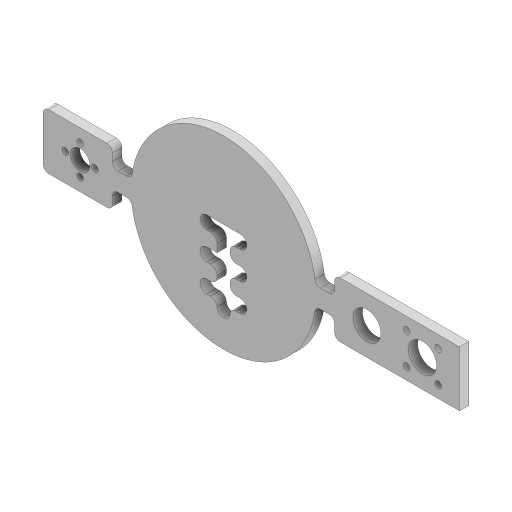
# Autodesk Inventor part: NUEVA TAPA PARA CORTE
Saved by Autodesk Inventor 2024 (Build 280153000, 153)
## iProperties
Created: 2024-05-26
Part Number: NUEVA TAPA PARA CORTE
Material: Generic
Document SubType Name: Modeling
Designer: Jhuliams
Density: 1 g/cm^3
Appearance: Default
Author: Jhuliams
Autodesk Inventor part; units mm, degrees
ref_plane "YZ Plane" through (0, 0, 0) normal (1, 0, 0) x (0, 1, 0)
ref_plane "XZ Plane" through (0, 0, 0) normal (0, 1, 0) x (-1, 0, 0)
ref_plane "XY Plane" through (0, 0, 0) normal (0, 0, 1) x (1, 0, 0)
sketch "Sketch1" plane through (0, 0, 0) normal (0, 0, 1) x (1, 0, 0)
  circle A0 centre (0, 0) radius 50
  line L0 (0, 0) -> (0, 20) construction
  line L1 (2.5, 15) -> (97.5, 15)
  line L2 (97.5, 15) -> (97.5, -15)
  line L3 (97.5, -15) -> (2.5, -15)
  line L4 (2.5, -15) -> (2.5, 15)
  line L5 (2.5, 15) -> (97.5, -15) construction
  line L6 (97.5, 15) -> (2.5, -15) construction
  line L7 (40, 5) -> (60, 5)
  line L8 (60, 5) -> (60, -5)
  line L9 (60, -5) -> (40, -5)
  line L10 (40, -5) -> (40, 5)
  line L11 (40, 5) -> (60, -5) construction
  line L12 (60, 5) -> (40, -5) construction
  line L13 (60, 5) -> (60, 15)
  line L14 (60, -5) -> (60, -15)
  line L15 (-2.5, 15) -> (-97.5, 15)
  line L16 (-97.5, 15) -> (-97.5, -15)
  line L17 (-97.5, -15) -> (-2.5, -15)
  line L18 (-2.5, -15) -> (-2.5, 15)
  line L19 (-2.5, 15) -> (-97.5, -15) construction
  line L20 (-97.5, 15) -> (-2.5, -15) construction
  line L21 (-40, 5) -> (-60, 5)
  line L22 (-60, 5) -> (-60, -5)
  line L23 (-60, -5) -> (-40, -5)
  line L24 (-40, -5) -> (-40, 5)
  line L25 (-40, 5) -> (-60, -5) construction
  line L26 (-60, 5) -> (-40, -5) construction
  line L27 (-60, 5) -> (-60, 15)
  line L28 (-60, -5) -> (-60, -15)
  line L29 (97.5, 15) -> (127.5, 15)
  line L30 (127.5, 15) -> (127.5, -15)
  line L31 (127.5, -15) -> (97.5, -15)
  line L32 (97.5, -15) -> (97.5, 15)
  point P0 (50, 0)
  point P1 (50, 0)
  point P2 (-50, 0)
  point P3 (-50, 0)
  point P4 (49.7494, 5)
  point P5 (49.7494, -5)
  point P6 (-49.7494, -5)
  point P7 (-49.7494, 5)
  dimension "d0" = 100
  dimension "d3" = 20
  dimension "d17" = 95
  dimension "d18" = 30
  dimension "d19" = 20
  dimension "d20" = 10
  dimension "d81" = 30
  dimension "d82" = 30
  constraints: 66 end point, 12 symmetric about line, 6 parallel, 5 midpoint, 5 perpendicular, 4 point on line, 3 horizontal, 1 coincident, 1 vertical, 3 other
  measures "d3" distance of L0.start L0.end
  measures "d17" distance of L2.end L3.end
  measures "d18" distance of L1.end L2.end
  measures "d19" distance of L8.end L9.end
  measures "d20" distance of L7.end L8.end
  measures "d81" distance of L30.end L31.end
  measures "d82" distance of L29.end L30.end
extrude "Extrusion1" add sketch "Sketch1" along normal blind 5 contours A0 L9 L10 L7 | A0 L7 L8 L9 | L7 L10 L9 A0 L3 L4 L1 | L1 L4 L3 A0 L17 L18 L15 | L13 L1 L2 L3 L14 L8 | L15 L18 L17 A0 L23 L24 L21 | L21 L24 L23 A0 | A0 L23 L22 L21 | L27 L22 L28 L17 L16 L15 | L29 L30 L31 L2
sketch "Sketch2" plane through (0, 0, 5) normal (0, 0, 1) x (1, 0, 0)
  line L0 (0, 0) -> (-77.5, 0) construction
  circle A0 centre (-77.5, 0) radius 5.25
  line L1 (0, 0) -> (0, 20) construction
  circle A1 centre (-77.5, 0) radius 8
  circle A2 centre (-69.5, 0) radius 1.75
  circle A3 centre (-77.5, 8) radius 1.75
  circle A4 centre (-85.5, 0) radius 1.75
  circle A5 centre (-77.5, -8) radius 1.75
  line L2 (0, 0) -> (107.5, 0)
  line L3 (0, 0) -> (107.5, 0) construction
  line L4 (95, 12.5) -> (120, 12.5)
  line L5 (120, 12.5) -> (120, -12.5)
  line L6 (120, -12.5) -> (95, -12.5)
  line L7 (95, -12.5) -> (95, 12.5)
  line L8 (95, 12.5) -> (120, -12.5) construction
  line L9 (120, 12.5) -> (95, -12.5) construction
  circle A6 centre (107.5, 0) radius 12
  line L10 (95, -12.5) -> (120, 12.5)
  circle A7 centre (115.9853, 8.4853) radius 1.75
  circle A8 centre (99.0147, 8.4853) radius 1.75
  circle A9 centre (99.0147, -8.4853) radius 1.75
  circle A10 centre (115.9853, -8.4853) radius 1.75
  circle A11 centre (107.5, 0) radius 7.6
  line L11 (0, 0) -> (77.5, 0)
  circle A12 centre (77.5, 0) radius 7.5
  dimension "d26" = 16
  dimension "d74" = 24
  dimension "d6" = 77.5
  dimension "d7" = 10.5
  dimension "d8" = 20
  dimension "d27" = 3.5
  dimension "d30" = 360
  dimension "d70" = 107.5
  dimension "d71" = 0
  dimension "d72" = 25
  dimension "d73" = 25
  dimension "d75" = 3.5
  dimension "d78" = 360
  dimension "d80" = 15.2
  dimension "d83" = 77.5
  dimension "d84" = 15
  constraints: 24 end point, 11 centre point, 6 coincident, 4 horizontal, 4 point on line, 3 equal length, 2 midpoint, 1 collinear, 1 horizontal alignment, 1 perpendicular, 1 vertical, 23 other
  measures "d6" distance of L0.start L0.end
  measures "d7" diameter of A0
  measures "d8" distance of L0.start L1.end
  measures "d27" diameter of A2
  measures "d70" distance of L0.start L2.end
  measures "d71" distance between parallel lines of L2 L3
  measures "d72" distance of L5.end L6.end
  measures "d73" distance of L4.end L5.end
  measures "d75" diameter of A7
  measures "d80" diameter of A11
  measures "d83" distance of L0.start L11.end
  measures "d84" diameter of A12
extrude "Extrusion2" cut sketch "Sketch2" against normal blind 7 contours A0 | A1 A2 | A1 A2 | A3 A1 | A1 A3 | A5 A1 | A1 A5 | A4 A1 | A1 A4 | L2 A12 | L2 A12 | A11 L10 L2 | L2 L10 A11 | A8 A6 | A6 A8 | A9 L10 A6 | A6 L10 A9 | L10 A6 A9 | L10 A11 | L10 A9 A6 | A7 A6 L10 | L10 A6 A7 | A7 A6 L10 | L10 A6 A7 | A10 A6 | A6 A10
fillet "Fillet1" radius 3 14 edges at (-60, 5, 2.5) (-60, 15, 2.5) (-49.7494, 5, 2.5) (-60, -5, 2.5) (-60, -15, 2.5) (-49.7494, -5, 2.5) (-97.5, -15, 2.5) (-97.5, 15, 2.5) (60, -15, 2.5) (60, 15, 2.5) (60, -5, 2.5) (60, 5, 2.5) (49.7494, 5, 2.5) (49.7494, -5, 2.5)
sketch "Sketch4" plane through (0, 0, 5) normal (0, 0, 1) x (1, 0, 0)
  line L0 (-3.5, 35) -> (3.5, 35)
  line L1 (3.5, 35) -> (3.5, -35)
  line L2 (3.5, -35) -> (-3.5, -35)
  line L3 (-3.5, -35) -> (-3.5, 35)
  line L4 (-3.5, 35) -> (3.5, -35) construction
  line L5 (3.5, 35) -> (-3.5, -35) construction
  line L6 (0, 0) -> (0, -25)
  line L7 (0, 0) -> (0, -10)
  line L8 (-12.5, -21.5) -> (12.5, -21.5)
  line L9 (12.5, -21.5) -> (12.5, -28.5)
  line L10 (12.5, -28.5) -> (-12.5, -28.5)
  line L11 (-12.5, -28.5) -> (-12.5, -21.5)
  line L12 (-12.5, -21.5) -> (12.5, -28.5) construction
  line L13 (12.5, -21.5) -> (-12.5, -28.5) construction
  line L14 (-12.5, -6.5) -> (12.5, -6.5)
  line L15 (12.5, -6.5) -> (12.5, -13.5)
  line L16 (12.5, -13.5) -> (-12.5, -13.5)
  line L17 (-12.5, -13.5) -> (-12.5, -6.5)
  line L18 (-12.5, -6.5) -> (12.5, -13.5) construction
  line L19 (12.5, -6.5) -> (-12.5, -13.5) construction
  line L20 (0, 0) -> (0, 5)
  line L21 (-12.5, 8.5) -> (12.5, 8.5)
  line L22 (12.5, 8.5) -> (12.5, 1.5)
  line L23 (12.5, 1.5) -> (-12.5, 1.5)
  line L24 (-12.5, 1.5) -> (-12.5, 8.5)
  line L25 (-12.5, 8.5) -> (12.5, 1.5) construction
  line L26 (12.5, 8.5) -> (-12.5, 1.5) construction
  point P0 (3.5, -21.5)
  point P1 (3.5, -13.5)
  point P2 (3.5, -6.5)
  point P3 (-3.5, -6.5)
  point P4 (-3.5, -13.5)
  point P5 (-3.5, -21.5)
  point P6 (-3.5, -28.5)
  point P7 (3.5, -28.5)
  point P8 (3.5, 8.5)
  point P9 (3.5, 1.5)
  point P10 (-3.5, 1.5)
  point P11 (-3.5, 8.5)
  dimension "d85" = 7
  dimension "d86" = 70
  dimension "d87" = 25
  dimension "d88" = 10
  dimension "d89" = 25
  dimension "d90" = 7
  dimension "d91" = 25
  dimension "d92" = 7
  dimension "d93" = 5
  dimension "d94" = 25
  dimension "d95" = 7
  constraints: 54 end point, 8 midpoint, 8 parallel, 4 horizontal, 4 perpendicular, 2 vertical, 1 point on line
  measures "d85" distance of L1.end L2.end
  measures "d86" distance of L0.end L1.end
  measures "d87" distance of L6.start L6.end
  measures "d88" distance of L6.start L7.end
  measures "d89" distance of L9.end L10.end
  measures "d90" distance of L8.end L9.end
  measures "d91" distance of L15.end L16.end
  measures "d92" distance of L14.end L15.end
  measures "d93" distance of L6.start L20.end
  measures "d94" distance of L22.end L23.end
  measures "d95" distance of L21.end L22.end
extrude "Extrusion3" cut sketch "Sketch4" against normal blind 10 contours L21 L1 L23 L3 | L3 L23 L24 L21 | L21 L22 L23 L1 | L23 L20 L6 L14 L3 | L1 L14 L6 L20 L23 | L14 L6 L16 L3 | L3 L16 L17 L14 | L14 L15 L16 L1 | L1 L16 L6 L14 | L16 L6 L8 L3 | L1 L8 L6 L16 | L8 L1 L10 L3 | L3 L10 L11 L8 | L8 L9 L10 L1 | L10 L1 L2 L3
fillet "Fillet2" radius 3.5 23 edges at (-12.5, 1.5, 2.5) (-12.5, -13.5, 2.5) (-12.5, -6.5, 2.5) (-12.5, 8.5, 2.5) (-12.5, -28.5, 2.5) (-12.5, -21.5, 2.5) (-3.5, -21.5, 2.5) (-3.5, -28.5, 2.5) (-3.5, -35, 2.5) (3.5, -35, 2.5) (3.5, -28.5, 2.5) (12.5, -28.5, 2.5) (12.5, -21.5, 2.5) (3.5, -21.5, 2.5) (-3.5, -13.5, 2.5) (-3.5, 1.5, 2.5) (3.5, -13.5, 2.5) (12.5, -13.5, 2.5) (12.5, 1.5, 2.5) (3.5, 1.5, 2.5) (3.5, -6.5, 2.5) (12.5, 8.5, 2.5) (12.5, -6.5, 2.5)
body "Solid1"
